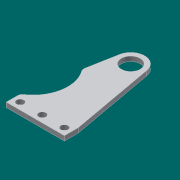
# Autodesk Inventor part: 足裏_メインフレーム_1_2
Saved by Autodesk Inventor 2016 (Build 200138000, 138)
## iProperties
Created: 2016-05-01
Part Number: 足裏_メインフレーム_1_2
Material: アルミニウム 2014-T4
Document SubType Name: Modeling
Designer: hiroaki
Density: 2.8 g/cm^3
Appearance: サテン
Mass: 3.9158 g
Surface Area: 17.6756 cm^2
Volume: 1.3985 cm^3
Author: hiroaki
Autodesk Inventor part; units mm, degrees
ref_plane "YZ Plane" through (0, 0, 0) normal (1, 0, 0) x (0, 1, 0)
ref_plane "XZ Plane" through (0, 0, 0) normal (0, 1, 0) x (-1, 0, 0)
ref_plane "XY Plane" through (0, 0, 0) normal (0, 0, 1) x (1, 0, 0)
derived "足裏_基礎_1.ipt"
sketch "スケッチ1" plane through (0, 0, 0) normal (0, 0, 1) x (1, 0, 0)
  circle A0 centre (0, 0) radius 5.05 construction
  line L0 (-21.25, 26.6) -> (21.25, 26.6) construction
  line L1 (21.25, 26.6) -> (21.25, -16) construction
  line L2 (21.25, -16) -> (-21.25, -16) construction
  line L3 (-21.25, -16) -> (-21.25, 26.6) construction
  circle A1 centre (0, 0) radius 26.6 construction
  line L4 (-12.5, -41) -> (12.5, -41) construction
  line L5 (12.5, -41) -> (12.5, -35) construction
  line L6 (12.5, -35) -> (10.99, 0.4679) construction
  line L7 (-12.5, -41) -> (-12.5, -35) construction
  line L8 (-12.5, -35) -> (-10.99, 0.4679) construction
  arc A2 (10.99, 0.4679) -> (-10.99, 0.4679) centre (0, 0) ccw construction
  line L9 (12.5, -35) -> (-12.5, -35) construction
  circle A3 centre (0, 8.5) radius 1.35 construction
  circle A4 centre (0, 8.5) radius 2.5 construction
  circle A5 centre (-8.5, 0) radius 1.35 construction
  circle A6 centre (0, -8.5) radius 1.35 construction
  circle A7 centre (8.5, 0) radius 1.35 construction
  circle A8 centre (-9.5, -38) radius 1.55
  circle A9 centre (0, -38) radius 1.55
  circle A10 centre (9.5, -38) radius 1.55
  line L10 (-12.5, -38) -> (12.5, -38) construction
  line L11 (0, 0) -> (0, -35) construction
  circle A11 centre (0, 0) radius 4.05
  circle A12 centre (0, 0) radius 6 construction
  line L12 (-12.5, -35) -> (-12.5, -41)
  line L13 (-12.5, -41) -> (12.5, -41)
  line L14 (12.5, -41) -> (12.5, -35)
  line L15 (12.5, -35) -> (5.9021, 1.0793)
  line L16 (-12.5, -35) -> (-5.9021, 1.0793)
  arc A13 (5.9021, 1.0793) -> (-5.9021, 1.0793) centre (0, 0) ccw
  line L17 (-6.3, -35) -> (-3.2, -35) construction
  line L18 (-3.2, -35) -> (-3.2, -41) construction
  line L19 (-3.2, -41) -> (-6.3, -41) construction
  line L20 (-6.3, -41) -> (-6.3, -35) construction
  line L21 (3.2, -35) -> (6.3, -35) construction
  line L22 (6.3, -35) -> (6.3, -41) construction
  line L23 (6.3, -41) -> (3.2, -41) construction
  line L24 (3.2, -41) -> (3.2, -35) construction
  line L25 (-4.75, -35) -> (-4.75, -41) construction
  line L26 (4.75, -35) -> (4.75, -41) construction
  point P0 (0, 26.6)
  point P1 (0, -41)
  dimension "d1" = 8.1
  dimension "d2" = 12
  measures "d1" diameter of A11
  measures "d2" diameter of A12
extrude "押し出し1" add sketch "スケッチ1" along normal blind 2
sketch "スケッチ3" plane through (-12.5, -41, 2) normal (0, 0, 1) x (1, 0, 0)
  circle A0 centre (12.5, 41) radius 4.05 projected
  line L0 (6.5979, 42.0793) -> (0, 6) projected
  arc A1 (0, 6) -> (4.112, 28.4857) centre (-7.5, 18.9904) ccw
  dimension "d5" = 15
  dimension "d6" = 20
  constraints: 2 point on circle, 1 centre point, 1 point on line
  measures "d5" radius of A1
  measures "d6" horizontal distance of A0.centre A1.centre
extrude "押し出し2" cut sketch "スケッチ3" against normal blind 10 contours A1 L0
fillet "フィレット1" radius 2 2 edges at (-8.388, -12.5143, 1) (-12.5, -35, 1)
